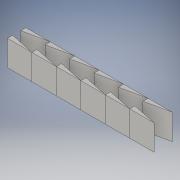
# Autodesk Inventor part: SawTeeth
Saved by Autodesk Inventor 2016 (Build 200138000, 138)
## iProperties
Created: 2016-03-05
Part Number: SawTeeth
Material: Generic
Document SubType Name: Modeling
Designer: yash
Density: 1 g/cm^3
Appearance: Default
Author: yash
Autodesk Inventor part; units mm, degrees
ref_plane "YZ Plane" through (0, 0, 0) normal (1, 0, 0) x (0, 1, 0)
ref_plane "XZ Plane" through (0, 0, 0) normal (0, 1, 0) x (-1, 0, 0)
ref_plane "XY Plane" through (0, 0, 0) normal (0, 0, 1) x (1, 0, 0)
sketch "Sketch3" plane through (0, 0, 0) normal (0, 1, 0) x (-1, 0, 0)
  line L0 (0, 0) -> (3.7528, 0)
  line L1 (3.7528, 0) -> (3.7528, -0.7937)
  line L2 (3.7528, -0.7937) -> (0, 0)
  line L3 (0, 0) -> (0, -1.4111) construction
  line L4 (0, -1.4111) -> (30.0228, -1.4111) construction
  line L5 (0, -2.8222) -> (3.7528, -2.8222)
  line L6 (3.7528, -2.8222) -> (3.7528, -2.0285)
  line L7 (3.7528, -2.0285) -> (0, -2.8222)
  line L8 (7.512, 0) -> (7.512, -0.7937)
  line L9 (3.7592, 0) -> (7.512, 0)
  line L10 (7.512, -0.7937) -> (3.7592, 0)
  line L11 (7.512, -2.0285) -> (3.7592, -2.8222)
  line L12 (7.512, -2.8222) -> (7.512, -2.0285)
  line L13 (3.7592, -2.8222) -> (7.512, -2.8222)
  line L14 (11.2712, 0) -> (11.2712, -0.7937)
  line L15 (7.5184, 0) -> (11.2712, 0)
  line L16 (11.2712, -0.7937) -> (7.5184, 0)
  line L17 (11.2712, -2.0285) -> (7.5184, -2.8222)
  line L18 (11.2712, -2.8222) -> (11.2712, -2.0285)
  line L19 (7.5184, -2.8222) -> (11.2712, -2.8222)
  line L20 (15.0304, 0) -> (15.0304, -0.7937)
  line L21 (11.2776, 0) -> (15.0304, 0)
  line L22 (15.0304, -0.7937) -> (11.2776, 0)
  line L23 (15.0304, -2.0285) -> (11.2776, -2.8222)
  line L24 (15.0304, -2.8222) -> (15.0304, -2.0285)
  line L25 (11.2776, -2.8222) -> (15.0304, -2.8222)
  line L26 (18.7897, 0) -> (18.7897, -0.7937)
  line L27 (15.0368, 0) -> (18.7897, 0)
  line L28 (18.7897, -0.7937) -> (15.0368, 0)
  line L29 (18.7897, -2.0285) -> (15.0368, -2.8222)
  line L30 (18.7897, -2.8222) -> (18.7897, -2.0285)
  line L31 (15.0368, -2.8222) -> (18.7897, -2.8222)
  line L32 (22.5488, 0) -> (22.5488, -0.7937)
  line L33 (18.796, 0) -> (22.5488, 0)
  line L34 (22.5488, -0.7937) -> (18.796, 0)
  line L35 (22.5488, -2.0285) -> (18.796, -2.8222)
  line L36 (22.5488, -2.8222) -> (22.5488, -2.0285)
  line L37 (18.796, -2.8222) -> (22.5488, -2.8222)
  dimension "d34" = 3.7529
  dimension "d35" = 0.7937
  dimension "d36" = 1.4111
  dimension "d37" = 30.0228
  dimension "d40" = 3.7592
  constraints: 76 end point, 3 symmetric about line, 2 horizontal, 2 vertical, 1 perpendicular, 60 other
  measures "d34" distance of L0.start L0.end
  measures "d35" distance of L0.end L1.end
  measures "d36" distance of L0.start L3.end
  measures "d37" distance of L3.end L4.end
  measures "d40" distance of L0.end L8.start
extrude "Extrusion2" add sketch "Sketch3" along normal blind 3.9116
body "Solid2"
